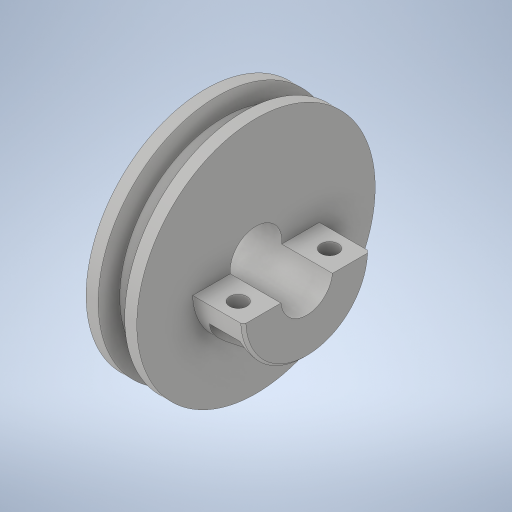
# Autodesk Inventor part: MBRDAC45-2-10_p1
Saved by Autodesk Inventor 2024 (Build 280153000, 153)
## iProperties
Created: 2024-03-05
Part Number: MBRDAC45-2-10_p1
Material: Generic
Catalog Web Link: www.cadenas.de
Description: MBRDC, MBRDAC_part1-Pulleys for Round Belts - Clamping Type - Trapezoid Groove
Vendor: MISUMI
Document SubType Name: Modeling
Designer: psAdmin
Manufacturer: MISUMI
Mass: 16.746 g
Surface Area: 63.6928 cm^2
Volume: 16.746 cm^3
Density: 1 g/cm^3
Appearance: PSOLRGB-175-175-175
Category: PARTsolutions
Company: MISUMI
PSOL_IDENT_0: {$CADENAS_DATA/23d-libs/misumi/metric/52_belts_pulleys/mbrdc/mbrdc_part1.prj},203 {VTYP=3D},{NB=MBRD
PSOL_IDENT_1: AC45-2-10_p1},{LINA=MBRDAC45-2-10},{NN=MBRDC, MBRDAC_part1},{DATE=01.02.2024 02:38:37},{GEOMDATE=19.
PSOL_IDENT_2: 01.2024 06:52:40},{VERSION=},{LINEID=30},{WBVAR=MAT,PD,DDS,ALT1},{WBNUMERIC=PD,DDS}  {NB=MBRDAC45-2-
PSOL_IDENT_3: 10_p1},{LINA=MBRDAC45-2-10},{KT=DUMMY},{PN=MBRDAC45-2-10},{TYPE=MBRDAC},{MAT=2},{ST=Clear Anodizing}
PSOL_IDENT_4: ,{AC=Hexagon Socket Head Cap Screw (x2) Stainless Steel},{PD=45},{PD0=23,28,30,40,45,48,60,80},{U=2.
PSOL_IDENT_5: 0},{DDS=10.00},{DS0=5,6,6.35,8,10,11,12},{D=25},{D1=47},{D2=41},{HH=2.0},{W=4.4},{L=20},{T=10},{LL=4
PSOL_IDENT_6: .5},{X=9.0},{Y=4.5},{M=M4},{CBD=4},{MM=4.000},{MMMIN=3.242},{DD1=8.0},{DD2=4.5},{ALT1=},{ALT1ALG='','
PSOL_IDENT_7: w/o DC (Outer Diameter Cut)','-DC','with DC (Outer Diameter Cut)'},{DC=0.0}
NB: MBRDAC45-2-10_p1
NN: MBRDC, MBRDAC_part1
NT: Pulleys for Round Belts - Clamping Type - Trapezoid Groove
NBSYN: $PN._p1
LINA: MBRDAC45-2-10
CATALOG: Misumi
PN: MBRDAC45-2-10
TYPE: MBRDAC
MAT: 5052 Aluminum Alloy
ST: Clear Anodizing
AC: Hexagon Socket Head Cap Screw (x2) Stainless Steel
PD: 45
U: 2
DDS: 10
D: 25
D1: 47
D2: 41
HH: 2
W: 4.4
L: 20
T: 10
LL: 4.5
X: 9
Y: 4.5
M: M4
CBD: 4
DD1: 8
DD2: 4.5
ALT1: w/o DC (Outer Diameter Cut)
DC: 0
SUPPLIER: MISUMI
ARTICLENO: MBRDAC45-2-10_p1
BOMINFO: MBRDAC45-2-10
CREATOR: CADENAS GmbH
Title: MBRDAC45-2-10
Author: Cadenas PARTsolutions
Comments: Pulleys for Round Belts - Clamping Type - Trapezoid Groove
Autodesk Inventor part; units mm, degrees
sketch "Sketch_1" plane through (0, 0, 0) normal (0, 0, 1) x (1, 0, 0)
  line L0 (5, 0) -> (-5, 0)
  line L1 (-5, 0) -> (-5, 23.5)
  line L2 (-5, 23.5) -> (-2.6142, 23.5)
  line L3 (-2.6142, 23.5) -> (-1.3716, 20.5)
  line L4 (-1.3716, 20.5) -> (1.3716, 20.5)
  line L5 (1.3716, 20.5) -> (2.6142, 23.5)
  line L6 (2.6142, 23.5) -> (5, 23.5)
  line L7 (5, 23.5) -> (5, 0)
  line L8 (5, 0) -> (-5, 0)
  constraints: 18 end point
revolve "Revolution1" add sketch "Sketch_1" angle 360 about axis through (5, 0, 0) along (1, 0, 0)
sketch "Sketch_2" plane through (0, 0, 0) normal (0, 0, 1) x (1, 0, 0)
  line L0 (5, 0) -> (15, 0)
  line L1 (15, 0) -> (15, -12)
  line L2 (15, -12) -> (14.5, -12.5)
  line L3 (14.5, -12.5) -> (5, -12.5)
  line L4 (5, -12.5) -> (5, 0)
  line L5 (5, 0) -> (15, 0)
  constraints: 12 end point
revolve "Revolution2" add sketch "Sketch_2" angle 180 mid plane about axis through (5, 0, 0) along (1, 0, 0)
sketch "Sketch_3" plane through (0, 0, 0) normal (0, 0, 1) x (1, 0, 0)
  line L0 (5, -0.5) -> (15, -0.5)
  line L1 (15, -0.5) -> (15, 0)
  line L2 (15, 0) -> (5, 0)
  line L3 (5, 0) -> (5, -0.5)
  constraints: 8 end point
extrude "Extrusion1" cut sketch "Sketch_3" along normal mid plane 50
sketch "Sketch_9" plane through (10.5, 0, 0) normal (1, 0, 0) x (0, 0, -1)
  line L0 (9, -12.5) -> (9, -0.5)
  line L1 (9, -0.5) -> (11, -0.5)
  line L2 (11, -0.5) -> (10.621, -0.879)
  line L3 (10.621, -0.879) -> (10.621, -12.121)
  line L4 (10.621, -12.121) -> (11, -12.5)
  line L5 (11, -12.5) -> (9, -12.5)
  line L6 (9, -12.5) -> (9, -0.5)
  constraints: 14 end point
sketch "Sketch_6" plane through (10.5, 0, 0) normal (1, 0, 0) x (0, 0, -1)
  line L0 (-9, -12.5) -> (-9, -0.5)
  line L1 (-9, -0.5) -> (-7, -0.5)
  line L2 (-7, -0.5) -> (-7.379, -0.879)
  line L3 (-7.379, -0.879) -> (-7.379, -12.121)
  line L4 (-7.379, -12.121) -> (-7, -12.5)
  line L5 (-7, -12.5) -> (-9, -12.5)
  line L6 (-9, -12.5) -> (-9, -0.5)
  constraints: 14 end point
ref_plane "part1_to_part2_XY" through (5, 0, 0) normal (1, 0, 0) x (0, 0, -1)
ref_plane "part1_to_part2_YZ" through (5, 0, 0) normal (0, 0, -1) x (0, 1, 0)
ref_plane "part1_to_part2_ZX" through (5, 0, 0) normal (0, 1, 0) x (1, 0, 0)
sketch "スケッチ7" plane through (5, -0.5, 12.49) normal (0, 1, 0) x (1, 0, 0)
  circle A0 centre (5.5, 3.49) radius 2 projected
  circle A1 centre (5.5, 3.49) radius 1.7
  circle A2 centre (5.5, 21.49) radius 2 projected
  circle A3 centre (5.5, 21.49) radius 1.7
  point P0 (-5, 12.49)
  dimension "d12" = 3.4
  dimension "d13" = 3.4
  constraints: 2 centre point, 2 coincident
  measures "d12" diameter of A1
  measures "d13" diameter of A3
hole "穴1" at (10.5, -0.5, 9) at (10.5, -0.5, -9) direction (0, -1, 0) diameter 3.4 end through all
sketch "スケッチ8" plane through (-5, 0, 0) normal (-1, 0, 0) x (0, 0, 1)
  point P0 (0, 0)
  point P1 (0, 0)
  constraints: 1 coincident
hole "穴2" at (-5, 0, 0) direction (1, 0, 0) diameter 10.2 end through all
ref_plane "作業平面4" through (9.75, -12.5, 0) normal (0, 1, 0) x (-1, 0, 0)
sketch "スケッチ9" plane through (9.75, -12.5, 0) normal (0, 1, 0) x (-1, 0, 0)
  circle A0 centre (-0.75, -9) radius 1.7 projected
  circle A1 centre (-0.75, -9) radius 4
  circle A2 centre (-0.75, 9) radius 1.7 projected
  circle A3 centre (-0.75, 9) radius 4
  point P0 (9.75, 0)
  dimension "d30" = 8
  dimension "d31" = 8
  constraints: 2 centre point, 2 coincident
  measures "d30" diameter of A1
  measures "d31" diameter of A3
extrude "押し出し2" cut sketch "スケッチ9" along normal blind 8 contours A0 | A1 | A3
body "Solid1"
